Autodesk Fusion 360 part; units mm, degrees
(part 6 of 15)
  spline S62 degree 5 poles (-42.8106, 4.7487) (-42.8188, 4.7555) (-42.8407, 4.7736) (-42.8766, 4.8029) (-42.9264, 4.8435) (-42.9903, 4.8952) (-43.0603, 4.9512) (-43.1305, 5.0069) (-43.2011, 5.0623) (-43.2719, 5.1174) (-43.3431, 5.1723) (-43.4145, 5.2269) (-43.4863, 5.2813) (-43.5583, 5.3354) (-43.6306, 5.3892) (-43.7031, 5.4428) (-43.776, 5.4962) (-43.8491, 5.5492) (-43.9224, 5.6021) (-43.9961, 5.6546) (-44.07, 5.707) (-44.1441, 5.7591) (-44.2185, 5.8109) (-44.2932, 5.8625) (-44.3681, 5.9139) (-44.4432, 5.965) (-44.5186, 6.0159) (-44.5942, 6.0665) (-44.6701, 6.1169) (-44.7462, 6.1671) (-44.8225, 6.2171) (-44.8991, 6.2668) (-44.9758, 6.3163) (-45.0529, 6.3656) (-45.1301, 6.4146) (-45.2075, 6.4634) (-45.2852, 6.512) (-45.3631, 6.5604) (-45.4412, 6.6085) (-45.5196, 6.6564) (-45.5981, 6.7041) (-45.6769, 6.7516) (-45.7558, 6.7988) (-45.8191, 6.8365) (-45.8667, 6.8646) (-45.8985, 6.8833) (-45.9144, 6.8927) knots 0.405839 0.405839 0.405839 0.405839 0.405839 0.405839 0.414286 0.428571 0.442857 0.457143 0.471429 0.485714 0.5 0.514286 0.528571 0.542857 0.557143 0.571429 0.585714 0.6 0.614286 0.628571 0.642857 0.657143 0.671429 0.685714 0.7 0.714286 0.728571 0.742857 0.757143 0.771429 0.785714 0.8 0.814286 0.828571 0.842857 0.857143 0.871429 0.885714 0.9 0.914286 0.928571 0.942857 0.957143 0.971429 0.985714 1 1 1 1 1 1
  arc A63 (-45.9144, 6.8927) -> (-46.9733, 6.0999) centre (-2.0032, -52.8695) ccw
  spline S63 degree 5 poles (-46.9733, 6.0999) (-46.9689, 6.0821) (-46.9599, 6.0463) (-46.9463, 5.9927) (-46.928, 5.9213) (-46.9049, 5.8323) (-46.8816, 5.7433) (-46.8579, 5.6545) (-46.834, 5.5659) (-46.8098, 5.4774) (-46.7854, 5.389) (-46.7606, 5.3008) (-46.7356, 5.2127) (-46.7103, 5.1248) (-46.6848, 5.037) (-46.6589, 4.9494) (-46.6328, 4.8619) (-46.6063, 4.7746) (-46.5796, 4.6875) (-46.5526, 4.6005) (-46.5253, 4.5136) (-46.4977, 4.427) (-46.4699, 4.3405) (-46.4417, 4.2541) (-46.4132, 4.168) (-46.3844, 4.082) (-46.3553, 3.9962) (-46.3259, 3.9105) (-46.2962, 3.8251) (-46.2662, 3.7398) (-46.2359, 3.6547) (-46.2052, 3.5698) (-46.1743, 3.485) (-46.143, 3.4005) (-46.1114, 3.3162) (-46.0794, 3.232) (-46.0471, 3.1481) (-46.0145, 3.0644) (-45.9816, 2.9808) (-45.9483, 2.8975) (-45.9146, 2.8144) (-45.8806, 2.7315) (-45.849, 2.6556) (-45.8241, 2.5964) (-45.806, 2.5537) (-45.7949, 2.5276) (-45.7907, 2.5179) knots -1 -1 -1 -1 -1 -1 -0.985714 -0.971429 -0.957143 -0.942857 -0.928571 -0.914286 -0.9 -0.885714 -0.871429 -0.857143 -0.842857 -0.828571 -0.814286 -0.8 -0.785714 -0.771429 -0.757143 -0.742857 -0.728571 -0.714286 -0.7 -0.685714 -0.671429 -0.657143 -0.642857 -0.628571 -0.614286 -0.6 -0.585714 -0.571429 -0.557143 -0.542857 -0.528571 -0.514286 -0.5 -0.485714 -0.471429 -0.457143 -0.442857 -0.428571 -0.414286 -0.405839 -0.405839 -0.405839 -0.405839 -0.405839 -0.405839
  arc A64 (-45.7907, 2.5179) -> (-46.8171, 1.6908) centre (-2.0032, -52.8695) ccw
  spline S64 degree 5 poles (-46.8171, 1.6908) (-46.8257, 1.6969) (-46.8489, 1.7134) (-46.8867, 1.7401) (-46.9393, 1.7771) (-47.0068, 1.824) (-47.0805, 1.8749) (-47.1546, 1.9254) (-47.2289, 1.9757) (-47.3035, 2.0256) (-47.3784, 2.0753) (-47.4536, 2.1247) (-47.529, 2.1738) (-47.6047, 2.2226) (-47.6806, 2.2711) (-47.7568, 2.3194) (-47.8333, 2.3674) (-47.91, 2.4151) (-47.987, 2.4626) (-48.0641, 2.5098) (-48.1416, 2.5567) (-48.2193, 2.6034) (-48.2972, 2.6498) (-48.3753, 2.6959) (-48.4537, 2.7418) (-48.5323, 2.7874) (-48.6111, 2.8328) (-48.6901, 2.878) (-48.7694, 2.9228) (-48.8489, 2.9675) (-48.9286, 3.0118) (-49.0085, 3.056) (-49.0886, 3.0999) (-49.1689, 3.1435) (-49.2495, 3.1869) (-49.3302, 3.2301) (-49.4112, 3.273) (-49.4923, 3.3157) (-49.5737, 3.3581) (-49.6552, 3.4003) (-49.737, 3.4423) (-49.8189, 3.484) (-49.901, 3.5255) (-49.9669, 3.5586) (-50.0164, 3.5832) (-50.0494, 3.5996) (-50.0659, 3.6078) knots 0.405839 0.405839 0.405839 0.405839 0.405839 0.405839 0.414286 0.428571 0.442857 0.457143 0.471429 0.485714 0.5 0.514286 0.528571 0.542857 0.557143 0.571429 0.585714 0.6 0.614286 0.628571 0.642857 0.657143 0.671429 0.685714 0.7 0.714286 0.728571 0.742857 0.757143 0.771429 0.785714 0.8 0.814286 0.828571 0.842857 0.857143 0.871429 0.885714 0.9 0.914286 0.928571 0.942857 0.957143 0.971429 0.985714 1 1 1 1 1 1
  arc A65 (-50.0659, 3.6078) -> (-51.0656, 2.7416) centre (-2.0032, -52.8695) ccw
  spline S65 degree 5 poles (-51.0656, 2.7416) (-51.0598, 2.724) (-51.0483, 2.689) (-51.031, 2.6365) (-51.0077, 2.5666) (-50.9783, 2.4794) (-50.9486, 2.3924) (-50.9187, 2.3055) (-50.8885, 2.2188) (-50.8581, 2.1322) (-50.8274, 2.0458) (-50.7964, 1.9596) (-50.7652, 1.8735) (-50.7337, 1.7877) (-50.7019, 1.7019) (-50.6699, 1.6164) (-50.6376, 1.531) (-50.605, 1.4458) (-50.5721, 1.3608) (-50.539, 1.2759) (-50.5056, 1.1913) (-50.4719, 1.1068) (-50.4379, 1.0225) (-50.4036, 0.9384) (-50.3691, 0.8545) (-50.3342, 0.7708) (-50.2991, 0.6872) (-50.2636, 0.6039) (-50.2279, 0.5208) (-50.1919, 0.4379) (-50.1556, 0.3551) (-50.1189, 0.2726) (-50.082, 0.1903) (-50.0448, 0.1083) (-50.0072, 0.0264) (-49.9693, -0.0553) (-49.9312, -0.1367) (-49.8927, -0.2179) (-49.8538, -0.2988) (-49.8147, -0.3796) (-49.7752, -0.4601) (-49.7353, -0.5403) (-49.6985, -0.6138) (-49.6694, -0.6711) (-49.6483, -0.7123) (-49.6353, -0.7376) (-49.6305, -0.747) knots -1 -1 -1 -1 -1 -1 -0.985714 -0.971429 -0.957143 -0.942857 -0.928571 -0.914286 -0.9 -0.885714 -0.871429 -0.857143 -0.842857 -0.828571 -0.814286 -0.8 -0.785714 -0.771429 -0.757143 -0.742857 -0.728571 -0.714286 -0.7 -0.685714 -0.671429 -0.657143 -0.642857 -0.628571 -0.614286 -0.6 -0.585714 -0.571429 -0.557143 -0.542857 -0.528571 -0.514286 -0.5 -0.485714 -0.471429 -0.457143 -0.442857 -0.428571 -0.414286 -0.405839 -0.405839 -0.405839 -0.405839 -0.405839 -0.405839
  arc A66 (-49.6305, -0.747) -> (-50.5952, -1.6452) centre (-2.0032, -52.8695) ccw
  spline S66 degree 5 poles (-50.5952, -1.6452) (-50.6042, -1.6397) (-50.6285, -1.625) (-50.6682, -1.601) (-50.7232, -1.5679) (-50.7939, -1.5259) (-50.8711, -1.4804) (-50.9486, -1.4353) (-51.0263, -1.3904) (-51.1043, -1.3459) (-51.1825, -1.3017) (-51.261, -1.2578) (-51.3397, -1.2142) (-51.4187, -1.1709) (-51.4979, -1.1279) (-51.5774, -1.0852) (-51.6571, -1.0428) (-51.737, -1.0007) (-51.8171, -0.9588) (-51.8975, -0.9173) (-51.9781, -0.876) (-52.0589, -0.835) (-52.1399, -0.7942) (-52.2211, -0.7538) (-52.3026, -0.7136) (-52.3842, -0.6737) (-52.4661, -0.6341) (-52.5482, -0.5947) (-52.6304, -0.5556) (-52.7129, -0.5167) (-52.7955, -0.4782) (-52.8784, -0.4398) (-52.9615, -0.4018) (-53.0447, -0.364) (-53.1281, -0.3264) (-53.2117, -0.2891) (-53.2955, -0.2521) (-53.3795, -0.2153) (-53.4637, -0.1788) (-53.548, -0.1425) (-53.6326, -0.1065) (-53.7173, -0.0707) (-53.8022, -0.0351) (-53.8702, -0.0069) (-53.9213, 0.0142) (-53.9554, 0.0282) (-53.9725, 0.0351) knots 0.405839 0.405839 0.405839 0.405839 0.405839 0.405839 0.414286 0.428571 0.442857 0.457143 0.471429 0.485714 0.5 0.514286 0.528571 0.542857 0.557143 0.571429 0.585714 0.6 0.614286 0.628571 0.642857 0.657143 0.671429 0.685714 0.7 0.714286 0.728571 0.742857 0.757143 0.771429 0.785714 0.8 0.814286 0.828571 0.842857 0.857143 0.871429 0.885714 0.9 0.914286 0.928571 0.942857 0.957143 0.971429 0.985714 1 1 1 1 1 1
  arc A67 (-53.9725, 0.0351) -> (-54.9078, -0.9002) centre (-2.0032, -52.8695) ccw
  spline S67 degree 5 poles (-54.9078, -0.9002) (-54.9009, -0.9173) (-54.8869, -0.9514) (-54.8658, -1.0025) (-54.8376, -1.0705) (-54.802, -1.1554) (-54.7662, -1.2401) (-54.7302, -1.3246) (-54.6939, -1.409) (-54.6574, -1.4932) (-54.6206, -1.5772) (-54.5836, -1.661) (-54.5463, -1.7446) (-54.5087, -1.828) (-54.4709, -1.9112) (-54.4329, -1.9943) (-54.3945, -2.0771) (-54.356, -2.1598) (-54.3171, -2.2423) (-54.278, -2.3245) (-54.2386, -2.4066) (-54.199, -2.4885) (-54.1591, -2.5701) (-54.1189, -2.6515) (-54.0784, -2.7328) (-54.0377, -2.8138) (-53.9967, -2.8946) (-53.9554, -2.9752) (-53.9139, -3.0556) (-53.872, -3.1357) (-53.8299, -3.2156) (-53.7875, -3.2953) (-53.7448, -3.3748) (-53.7018, -3.454) (-53.6585, -3.533) (-53.6149, -3.6117) (-53.571, -3.6902) (-53.5268, -3.7684) (-53.4822, -3.8464) (-53.4374, -3.9241) (-53.3923, -4.0016) (-53.3468, -4.0788) (-53.3048, -4.1495) (-53.2717, -4.2045) (-53.2477, -4.2442) (-53.233, -4.2685) (-53.2275, -4.2775) knots -1 -1 -1 -1 -1 -1 -0.985714 -0.971429 -0.957143 -0.942857 -0.928571 -0.914286 -0.9 -0.885714 -0.871429 -0.857143 -0.842857 -0.828571 -0.814286 -0.8 -0.785714 -0.771429 -0.757143 -0.742857 -0.728571 -0.714286 -0.7 -0.685714 -0.671429 -0.657143 -0.642857 -0.628571 -0.614286 -0.6 -0.585714 -0.571429 -0.557143 -0.542857 -0.528571 -0.514286 -0.5 -0.485714 -0.471429 -0.457143 -0.442857 -0.428571 -0.414286 -0.405839 -0.405839 -0.405839 -0.405839 -0.405839 -0.405839
  arc A68 (-53.2275, -4.2775) -> (-54.1257, -5.2422) centre (-2.0032, -52.8695) ccw
  spline S68 degree 5 poles (-54.1257, -5.2422) (-54.1351, -5.2374) (-54.1604, -5.2244) (-54.2016, -5.2033) (-54.2589, -5.1742) (-54.3324, -5.1374) (-54.4126, -5.0975) (-54.4931, -5.058) (-54.5739, -5.0189) (-54.6548, -4.98) (-54.736, -4.9415) (-54.8174, -4.9033) (-54.8991, -4.8655) (-54.9809, -4.8279) (-55.063, -4.7907) (-55.1453, -4.7538) (-55.2278, -4.7171) (-55.3106, -4.6808) (-55.3935, -4.6448) (-55.4766, -4.6091) (-55.5599, -4.5736) (-55.6435, -4.5385) (-55.7272, -4.5036) (-55.8111, -4.4691) (-55.8952, -4.4348) (-55.9795, -4.4008) (-56.064, -4.3671) (-56.1486, -4.3337) (-56.2335, -4.3006) (-56.3185, -4.2677) (-56.4037, -4.2351) (-56.4891, -4.2028) (-56.5746, -4.1708) (-56.6603, -4.139) (-56.7462, -4.1075) (-56.8323, -4.0763) (-56.9185, -4.0453) (-57.0049, -4.0146) (-57.0915, -3.9842) (-57.1782, -3.954) (-57.2651, -3.9241) (-57.3521, -3.8944) (-57.4393, -3.865) (-57.5092, -3.8417) (-57.5617, -3.8244) (-57.5967, -3.8128) (-57.6143, -3.8071) knots 0.405839 0.405839 0.405839 0.405839 0.405839 0.405839 0.414286 0.428571 0.442857 0.457143 0.471429 0.485714 0.5 0.514286 0.528571 0.542857 0.557143 0.571429 0.585714 0.6 0.614286 0.628571 0.642857 0.657143 0.671429 0.685714 0.7 0.714286 0.728571 0.742857 0.757143 0.771429 0.785714 0.8 0.814286 0.828571 0.842857 0.857143 0.871429 0.885714 0.9 0.914286 0.928571 0.942857 0.957143 0.971429 0.985714 1 1 1 1 1 1
  arc A69 (-57.6143, -3.8071) -> (-58.4805, -4.8068) centre (-2.0032, -52.8695) ccw
  spline S69 degree 5 poles (-58.4805, -4.8068) (-58.4723, -4.8233) (-58.4559, -4.8563) (-58.4313, -4.9058) (-58.3982, -4.9717) (-58.3567, -5.0538) (-58.315, -5.1357) (-58.273, -5.2175) (-58.2308, -5.299) (-58.1884, -5.3804) (-58.1457, -5.4615) (-58.1028, -5.5425) (-58.0596, -5.6232) (-58.0162, -5.7037) (-57.9726, -5.7841) (-57.9287, -5.8642) (-57.8845, -5.9441) (-57.8402, -6.0238) (-57.7955, -6.1033) (-57.7507, -6.1826) (-57.7055, -6.2616) (-57.6601, -6.3404) (-57.6145, -6.419) (-57.5686, -6.4974) (-57.5225, -6.5755) (-57.4761, -6.6534) (-57.4294, -6.7311) (-57.3825, -6.8085) (-57.3353, -6.8857) (-57.2878, -6.9627) (-57.2401, -7.0394) (-57.1921, -7.1159) (-57.1438, -7.1921) (-57.0953, -7.268) (-57.0465, -7.3437) (-56.9974, -7.4191) (-56.948, -7.4943) (-56.8983, -7.5692) (-56.8484, -7.6438) (-56.7981, -7.7181) (-56.7476, -7.7922) (-56.6967, -7.8659) (-56.6497, -7.9334) (-56.6128, -7.986) (-56.5861, -8.0238) (-56.5696, -8.047) (-56.5635, -8.0556) knots -1 -1 -1 -1 -1 -1 -0.985714 -0.971429 -0.957143 -0.942857 -0.928571 -0.914286 -0.9 -0.885714 -0.871429 -0.857143 -0.842857 -0.828571 -0.814286 -0.8 -0.785714 -0.771429 -0.757143 -0.742857 -0.728571 -0.714286 -0.7 -0.685714 -0.671429 -0.657143 -0.642857 -0.628571 -0.614286 -0.6 -0.585714 -0.571429 -0.557143 -0.542857 -0.528571 -0.514286 -0.5 -0.485714 -0.471429 -0.457143 -0.442857 -0.428571 -0.414286 -0.405839 -0.405839 -0.405839 -0.405839 -0.405839 -0.405839
  arc A70 (-56.5635, -8.0556) -> (-57.3905, -9.082) centre (-2.0032, -52.8695) ccw
  spline S70 degree 5 poles (-57.3905, -9.082) (-57.4003, -9.0778) (-57.4264, -9.0667) (-57.4691, -9.0486) (-57.5283, -9.0236) (-57.6042, -8.9921) (-57.6871, -8.9581) (-57.7702, -8.9244) (-57.8535, -8.8911) (-57.9371, -8.8582) (-58.0208, -8.8256) (-58.1047, -8.7933) (-58.1889, -8.7613) (-58.2732, -8.7297) (-58.3577, -8.6984) (-58.4425, -8.6675) (-58.5274, -8.6368) (-58.6125, -8.6065) (-58.6978, -8.5765) (-58.7832, -8.5468) (-58.8689, -8.5174) (-58.9547, -8.4883) (-59.0407, -8.4595) (-59.1268, -8.431) (-59.2132, -8.4028) (-59.2997, -8.3749) (-59.3863, -8.3474) (-59.4732, -8.3201) (-59.5602, -8.2931) (-59.6473, -8.2664) (-59.7346, -8.2399) (-59.8221, -8.2138) (-59.9097, -8.1879) (-59.9975, -8.1624) (-60.0854, -8.1371) (-60.1735, -8.1121) (-60.2617, -8.0873) (-60.3501, -8.0629) (-60.4386, -8.0387) (-60.5272, -8.0148) (-60.616, -7.9911) (-60.705, -7.9678) (-60.794, -7.9447) (-60.8654, -7.9264) (-60.919, -7.9128) (-60.9548, -7.9038) (-60.9726, -7.8993) knots 0.405839 0.405839 0.405839 0.405839 0.405839 0.405839 0.414286 0.428571 0.442857 0.457143 0.471429 0.485714 0.5 0.514286 0.528571 0.542857 0.557143 0.571429 0.585714 0.6 0.614286 0.628571 0.642857 0.657143 0.671429 0.685714 0.7 0.714286 0.728571 0.742857 0.757143 0.771429 0.785714 0.8 0.814286 0.828571 0.842857 0.857143 0.871429 0.885714 0.9 0.914286 0.928571 0.942857 0.957143 0.971429 0.985714 1 1 1 1 1 1
  arc A71 (-60.9726, -7.8993) -> (-61.7653, -8.9583) centre (-2.0032, -52.8695) ccw
  spline S71 degree 5 poles (-61.7653, -8.9583) (-61.756, -8.9742) (-61.7373, -9.006) (-61.7092, -9.0535) (-61.6715, -9.1169) (-61.6243, -9.1958) (-61.5768, -9.2746) (-61.5291, -9.3531) (-61.4812, -9.4315) (-61.4331, -9.5096) (-61.3847, -9.5875) (-61.3361, -9.6651) (-61.2873, -9.7426) (-61.2383, -9.8198) (-61.189, -9.8969) (-61.1395, -9.9736) (-61.0898, -10.0502) (-61.0398, -10.1265) (-60.9896, -10.2026) (-60.9392, -10.2785) (-60.8886, -10.3541) (-60.8377, -10.4295) (-60.7866, -10.5046) (-60.7352, -10.5795) (-60.6836, -10.6542) (-60.6317, -10.7286) (-60.5797, -10.8027) (-60.5273, -10.8766) (-60.4747, -10.9502) (-60.4219, -11.0236) (-60.3688, -11.0967) (-60.3155, -11.1696) (-60.2619, -11.2421) (-60.2081, -11.3144) (-60.154, -11.3864) (-60.0996, -11.4582) (-60.045, -11.5296) (-59.9901, -11.6008) (-59.935, -11.6716) (-59.8795, -11.7422) (-59.8238, -11.8124) (-59.7679, -11.8824) (-59.7162, -11.9463) (-59.6756, -11.9961) (-59.6462, -12.032) (-59.6282, -12.0539) (-59.6214, -12.0621) knots -1 -1 -1 -1 -1 -1 -0.985714 -0.971429 -0.957143 -0.942857 -0.928571 -0.914286 -0.9 -0.885714 -0.871429 -0.857143 -0.842857 -0.828571 -0.814286 -0.8 -0.785714 -0.771429 -0.757143 -0.742857 -0.728571 -0.714286 -0.7 -0.685714 -0.671429 -0.657143 -0.642857 -0.628571 -0.614286 -0.6 -0.585714 -0.571429 -0.557143 -0.542857 -0.528571 -0.514286 -0.5 -0.485714 -0.471429 -0.457143 -0.442857 -0.428571 -0.414286 -0.405839 -0.405839 -0.405839 -0.405839 -0.405839 -0.405839
  arc A72 (-59.6214, -12.0621) -> (-60.3732, -13.1448) centre (-2.0032, -52.8695) ccw
  spline S72 degree 5 poles (-60.3732, -13.1448) (-60.3832, -13.1414) (-60.4101, -13.1321) (-60.4539, -13.1171) (-60.5148, -13.0965) (-60.5927, -13.0704) (-60.6778, -13.0424) (-60.7631, -13.0148) (-60.8486, -12.9875) (-60.9343, -12.9606) (-61.0201, -12.934) (-61.1062, -12.9078) (-61.1924, -12.882) (-61.2787, -12.8564) (-61.3653, -12.8313) (-61.452, -12.8064) (-61.5389, -12.7819) (-61.6259, -12.7577) (-61.7131, -12.7339) (-61.8005, -12.7103) (-61.888, -12.6871) (-61.9757, -12.6642) (-62.0635, -12.6417) (-62.1515, -12.6194) (-62.2396, -12.5974) (-62.3279, -12.5758) (-62.4163, -12.5545) (-62.5049, -12.5334) (-62.5936, -12.5127) (-62.6824, -12.4923) (-62.7714, -12.4721) (-62.8605, -12.4523) (-62.9497, -12.4328) (-63.0391, -12.4135) (-63.1286, -12.3946) (-63.2182, -12.3759) (-63.308, -12.3575) (-63.3979, -12.3394) (-63.4879, -12.3216) (-63.578, -12.3041) (-63.6683, -12.2869) (-63.7586, -12.2699) (-63.8491, -12.2532) (-63.9216, -12.2401) (-63.9761, -12.2304) (-64.0124, -12.224) (-64.0305, -12.2208) knots 0.405839 0.405839 0.405839 0.405839 0.405839 0.405839 0.414286 0.428571 0.442857 0.457143 0.471429 0.485714 0.5 0.514286 0.528571 0.542857 0.557143 0.571429 0.585714 0.6 0.614286 0.628571 0.642857 0.657143 0.671429 0.685714 0.7 0.714286 0.728571 0.742857 0.757143 0.771429 0.785714 0.8 0.814286 0.828571 0.842857 0.857143 0.871429 0.885714 0.9 0.914286 0.928571 0.942857 0.957143 0.971429 0.985714 1 1 1 1 1 1
  arc A73 (-64.0305, -12.2208) -> (-64.7457, -13.3335) centre (-2.0032, -52.8695) ccw
  spline S73 degree 5 poles (-64.7457, -13.3335) (-64.7352, -13.3487) (-64.7143, -13.3791) (-64.6828, -13.4246) (-64.6408, -13.485) (-64.588, -13.5604) (-64.535, -13.6356) (-64.4819, -13.7105) (-64.4285, -13.7852) (-64.3749, -13.8597) (-64.3211, -13.934) (-64.2671, -14.008) (-64.2129, -14.0818) (-64.1585, -14.1553) (-64.1038, -14.2286) (-64.049, -14.3017) (-63.9939, -14.3745) (-63.9386, -14.4471) (-63.8832, -14.5194) (-63.8275, -14.5914) (-63.7715, -14.6633) (-63.7154, -14.7348) (-63.6591, -14.8061) (-63.6025, -14.8772) (-63.5457, -14.9479) (-63.4887, -15.0185) (-63.4314, -15.0887) (-63.374, -15.1587) (-63.3163, -15.2284) (-63.2583, -15.2978) (-63.2002, -15.3669) (-63.1418, -15.4358) (-63.0832, -15.5043) (-63.0243, -15.5726) (-62.9652, -15.6406) (-62.9059, -15.7082) (-62.8463, -15.7756) (-62.7865, -15.8427) (-62.7264, -15.9094) (-62.6661, -15.9758) (-62.6055, -16.0419) (-62.5447, -16.1077) (-62.4886, -16.1678) (-62.4446, -16.2146) (-62.4127, -16.2482) (-62.3931, -16.2688) (-62.3858, -16.2765) knots -1 -1 -1 -1 -1 -1 -0.985714 -0.971429 -0.957143 -0.942857 -0.928571 -0.914286 -0.9 -0.885714 -0.871429 -0.857143 -0.842857 -0.828571 -0.814286 -0.8 -0.785714 -0.771429 -0.757143 -0.742857 -0.728571 -0.714286 -0.7 -0.685714 -0.671429 -0.657143 -0.642857 -0.628571 -0.614286 -0.6 -0.585714 -0.571429 -0.557143 -0.542857 -0.528571 -0.514286 -0.5 -0.485714 -0.471429 -0.457143 -0.442857 -0.428571 -0.414286 -0.405839 -0.405839 -0.405839 -0.405839 -0.405839 -0.405839
  arc A74 (-62.3858, -16.2765) -> (-63.0584, -17.4101) centre (-2.0032, -52.8695) ccw
  spline S74 degree 5 poles (-63.0584, -17.4101) (-63.0686, -17.4074) (-63.0961, -17.4) (-63.1409, -17.3882) (-63.2031, -17.372) (-63.2827, -17.3516) (-63.3696, -17.3297) (-63.4566, -17.3082) (-63.5438, -17.2871) (-63.6312, -17.2664) (-63.7187, -17.246) (-63.8064, -17.226) (-63.8942, -17.2063) (-63.9822, -17.1871) (-64.0703, -17.1681) (-64.1586, -17.1495) (-64.247, -17.1313) (-64.3356, -17.1134) (-64.4242, -17.0958) (-64.5131, -17.0785) (-64.602, -17.0616) (-64.6911, -17.0451) (-64.7803, -17.0288) (-64.8697, -17.0129) (-64.9591, -16.9973) (-65.0487, -16.982) (-65.1384, -16.967) (-65.2282, -16.9523) (-65.3182, -16.938) (-65.4083, -16.924) (-65.4984, -16.9102) (-65.5887, -16.8968) (-65.6791, -16.8837) (-65.7697, -16.8709) (-65.8603, -16.8583) (-65.951, -16.8461) (-66.0419, -16.8342) (-66.1328, -16.8226) (-66.2239, -16.8112) (-66.315, -16.8002) (-66.4063, -16.7894) (-66.4976, -16.7789) (-66.5891, -16.7687) (-66.6623, -16.7608) (-66.7173, -16.755) (-66.754, -16.7512) (-66.7723, -16.7493) knots 0.405839 0.405839 0.405839 0.405839 0.405839 0.405839 0.414286 0.428571 0.442857 0.457143 0.471429 0.485714 0.5 0.514286 0.528571 0.542857 0.557143 0.571429 0.585714 0.6 0.614286 0.628571 0.642857 0.657143 0.671429 0.685714 0.7 0.714286 0.728571 0.742857 0.757143 0.771429 0.785714 0.8 0.814286 0.828571 0.842857 0.857143 0.871429 0.885714 0.9 0.914286 0.928571 0.942857 0.957143 0.971429 0.985714 1 1 1 1 1 1
  arc A75 (-66.7723, -16.7493) -> (-67.4063, -17.9103) centre (-2.0032, -52.8695) ccw
  spline S75 degree 5 poles (-67.4063, -17.9103) (-67.3948, -17.9247) (-67.3717, -17.9535) (-67.3371, -17.9966) (-67.2908, -18.0539) (-67.2328, -18.1253) (-67.1746, -18.1965) (-67.1162, -18.2675) (-67.0577, -18.3382) (-66.9989, -18.4087) (-66.9399, -18.4789) (-66.8808, -18.5489) (-66.8215, -18.6186) (-66.7619, -18.6881) (-66.7022, -18.7573) (-66.6423, -18.8262) (-66.5822, -18.8949) (-66.5219, -18.9634) (-66.4614, -19.0316) (-66.4007, -19.0995) (-66.3398, -19.1671) (-66.2787, -19.2345) (-66.2174, -19.3016) (-66.1559, -19.3684) (-66.0942, -19.435) (-66.0323, -19.5012) (-65.9702, -19.5672) (-65.9078, -19.6329) (-65.8453, -19.6983) (-65.7826, -19.7634) (-65.7197, -19.8282) (-65.6565, -19.8927) (-65.5931, -19.9569) (-65.5296, -20.0208) (-65.4658, -20.0844) (-65.4017, -20.1477) (-65.3375, -20.2106) (-65.2731, -20.2732) (-65.2084, -20.3355) (-65.1435, -20.3975) (-65.0783, -20.4591) (-65.013, -20.5203) (-64.9528, -20.5763) (-64.9055, -20.6198) (-64.8713, -20.6511) (-64.8503, -20.6703) (-64.8425, -20.6774) knots -1 -1 -1 -1 -1 -1 -0.985714 -0.971429 -0.957143 -0.942857 -0.928571 -0.914286 -0.9 -0.885714 -0.871429 -0.857143 -0.842857 -0.828571 -0.814286 -0.8 -0.785714 -0.771429 -0.757143 -0.742857 -0.728571 -0.714286 -0.7 -0.685714 -0.671429 -0.657143 -0.642857 -0.628571 -0.614286 -0.6 -0.585714 -0.571429 -0.557143 -0.542857 -0.528571 -0.514286 -0.5 -0.485714 -0.471429 -0.457143 -0.442857 -0.428571 -0.414286 -0.405839 -0.405839 -0.405839 -0.405839 -0.405839 -0.405839
  arc A76 (-64.8425, -20.6774) -> (-65.4325, -21.8561) centre (-2.0032, -52.8695) ccw
  spline S76 degree 5 poles (-65.4325, -21.8561) (-65.4429, -21.8541) (-65.4708, -21.8487) (-65.5163, -21.8401) (-65.5795, -21.8284) (-65.6604, -21.8137) (-65.7486, -21.7981) (-65.837, -21.7829) (-65.9254, -21.768) (-66.0141, -21.7536) (-66.1028, -21.7395) (-66.1917, -21.7258) (-66.2807, -21.7125) (-66.3698, -21.6995) (-66.4591, -21.6869) (-66.5485, -21.6746) (-66.638, -21.6627) (-66.7276, -21.6512) (-66.8173, -21.64) (-66.9071, -21.6291) (-66.997, -21.6186) (-67.0871, -21.6084) (-67.1772, -21.5986) (-67.2675, -21.5891) (-67.3578, -21.5799) (-67.4483, -21.571) (-67.5388, -21.5625) (-67.6295, -21.5543) (-67.7202, -21.5464) (-67.811, -21.5388) (-67.902, -21.5315) (-67.993, -21.5246) (-68.0841, -21.518) (-68.1753, -21.5116) (-68.2666, -21.5056) (-68.358, -21.4999) (-68.4494, -21.4945) (-68.541, -21.4894) (-68.6326, -21.4845) (-68.7243, -21.48) (-68.8161, -21.4758) (-68.908, -21.4719) (-68.9999, -21.4682) (-69.0736, -21.4656) (-69.1288, -21.4637) (-69.1657, -21.4625) (-69.1841, -21.4619) knots 0.405839 0.405839 0.405839 0.405839 0.405839 0.405839 0.414286 0.428571 0.442857 0.457143 0.471429 0.485714 0.5 0.514286 0.528571 0.542857 0.557143 0.571429 0.585714 0.6 0.614286 0.628571 0.642857 0.657143 0.671429 0.685714 0.7 0.714286 0.728571 0.742857 0.757143 0.771429 0.785714 0.8 0.814286 0.828571 0.842857 0.857143 0.871429 0.885714 0.9 0.914286 0.928571 0.942857 0.957143 0.971429 0.985714 1 1 1 1 1 1
  arc A77 (-69.1841, -21.4619) -> (-69.7336, -22.6651) centre (-2.0032, -52.8695) ccw
  spline S77 degree 5 poles (-69.7336, -22.6651) (-69.7211, -22.6787) (-69.6961, -22.7058) (-69.6585, -22.7463) (-69.6082, -22.8002) (-69.5453, -22.8673) (-69.4821, -22.9341) (-69.4188, -23.0008) (-69.3553, -23.0671) (-69.2917, -23.1332) (-69.2279, -23.199) (-69.1639, -23.2646) (-69.0997, -23.3299) (-69.0354, -23.395) (-68.9709, -23.4598) (-68.9062, -23.5243) (-68.8414, -23.5885) (-68.7763, -23.6525) (-68.7111, -23.7162) (-68.6457, -23.7796) (-68.5801, -23.8427) (-68.5144, -23.9055) (-68.4485, -23.9681) (-68.3824, -24.0304) (-68.3161, -24.0923) (-68.2496, -24.154) (-68.1829, -24.2154) (-68.1161, -24.2765) (-68.0491, -24.3373) (-67.9818, -24.3977) (-67.9144, -24.4579) (-67.8469, -24.5177) (-67.7791, -24.5772) (-67.7111, -24.6364) (-67.6429, -24.6953) (-67.5746, -24.7538) (-67.506, -24.812) (-67.4372, -24.8699) (-67.3683, -24.9274) (-67.2991, -24.9846) (-67.2298, -25.0414) (-67.1602, -25.0978) (-67.0961, -25.1493) (-67.0459, -25.1894) (-67.0096, -25.2181) (-66.9872, -25.2358) (-66.9789, -25.2423) knots -1 -1 -1 -1 -1 -1 -0.985714 -0.971429 -0.957143 -0.942857 -0.928571 -0.914286 -0.9 -0.885714 -0.871429 -0.857143 -0.842857 -0.828571 -0.814286 -0.8 -0.785714 -0.771429 -0.757143 -0.742857 -0.728571 -0.714286 -0.7 -0.685714 -0.671429 -0.657143 -0.642857 -0.628571 -0.614286 -0.6 -0.585714 -0.571429 -0.557143 -0.542857 -0.528571 -0.514286 -0.5 -0.485714 -0.471429 -0.457143 -0.442857 -0.428571 -0.414286 -0.405839 -0.405839 -0.405839 -0.405839 -0.405839 -0.405839
  arc A78 (-66.9789, -25.2423) -> (-67.4833, -26.4601) centre (-2.0032, -52.8695) ccw
  spline S78 degree 5 poles (-67.4833, -26.4601) (-67.4938, -26.4588) (-67.5221, -26.4555) (-67.5681, -26.4502) (-67.632, -26.4429) (-67.7137, -26.4341) (-67.8028, -26.4248) (-67.892, -26.4159) (-67.9813, -26.4074) (-68.0708, -26.3993) (-68.1603, -26.3916) (-68.2499, -26.3843) (-68.3397, -26.3774) (-68.4295, -26.3708) (-68.5194, -26.3646) (-68.6094, -26.3587) (-68.6995, -26.3532) (-68.7897, -26.3481) (-68.88, -26.3433) (-68.9704, -26.3389) (-69.0608, -26.3348) (-69.1514, -26.3311) (-69.242, -26.3277) (-69.3327, -26.3247) (-69.4235, -26.322) (-69.5143, -26.3196) (-69.6052, -26.3175) (-69.6962, -26.3158) (-69.7873, -26.3144) (-69.8785, -26.3133) (-69.9697, -26.3126) (-70.061, -26.3121) (-70.1523, -26.312) (-70.2438, -26.3122) (-70.3352, -26.3127) (-70.4268, -26.3135) (-70.5184, -26.3146) (-70.6101, -26.3161) (-70.7018, -26.3178) (-70.7936, -26.3198) (-70.8855, -26.3222) (-70.9774, -26.3248) (-71.0694, -26.3277) (-71.143, -26.3303) (-71.1982, -26.3324) (-71.2351, -26.3338) (-71.2535, -26.3346) knots 0.405839 0.405839 0.405839 0.405839 0.405839 0.405839 0.414286 0.428571 0.442857 0.457143 0.471429 0.485714 0.5 0.514286 0.528571 0.542857 0.557143 0.571429 0.585714 0.6 0.614286 0.628571 0.642857 0.657143 0.671429 0.685714 0.7 0.714286 0.728571 0.742857 0.757143 0.771429 0.785714 0.8 0.814286 0.828571 0.842857 0.857143 0.871429 0.885714 0.9 0.914286 0.928571 0.942857 0.957143 0.971429 0.985714 1 1 1 1 1 1
  arc A79 (-71.2535, -26.3346) -> (-71.7158, -27.5739) centre (-2.0032, -52.8695) ccw
  spline S79 degree 5 poles (-71.7158, -27.5739) (-71.7023, -27.5866) (-71.6754, -27.6118) (-71.635, -27.6495) (-71.5811, -27.6997) (-71.5135, -27.7621) (-71.4458, -27.8243) (-71.3779, -27.8862) (-71.3098, -27.9479) (-71.2416, -28.0093) (-71.1733, -28.0704) (-71.1048, -28.1312) (-71.0361, -28.1918) (-70.9673, -28.2521) (-70.8983, -28.3121) (-70.8292, -28.3718) (-70.7599, -28.4313) (-70.6905, -28.4905) (-70.6209, -28.5493) (-70.5512, -28.6079) (-70.4813, -28.6662) (-70.4112, -28.7242) (-70.341, -28.7819) (-70.2706, -28.8393) (-70.2, -28.8964) (-70.1293, -28.9531) (-70.0585, -29.0096) (-69.9874, -29.0658) (-69.9163, -29.1216) (-69.8449, -29.1771) (-69.7734, -29.2323) (-69.7017, -29.2872) (-69.6298, -29.3417) (-69.5578, -29.3959) (-69.4856, -29.4498) (-69.4132, -29.5033) (-69.3407, -29.5564) (-69.268, -29.6092) (-69.1951, -29.6617) (-69.1221, -29.7138) (-69.0488, -29.7655) (-68.9754, -29.8168) (-68.9078, -29.8636) (-68.8548, -29.9) (-68.8166, -29.9261) (-68.793, -29.9421) (-68.7843, -29.948) knots -1 -1 -1 -1 -1 -1 -0.985714 -0.971429 -0.957143 -0.942857 -0.928571 -0.914286 -0.9 -0.885714 -0.871429 -0.857143 -0.842857 -0.828571 -0.814286 -0.8 -0.785714 -0.771429 -0.757143 -0.742857 -0.728571 -0.714286 -0.7 -0.685714 -0.671429 -0.657143 -0.642857 -0.628571 -0.614286 -0.6 -0.585714 -0.571429 -0.557143 -0.542857 -0.528571 -0.514286 -0.5 -0.485714 -0.471429 -0.457143 -0.442857 -0.428571 -0.414286 -0.405839 -0.405839 -0.405839 -0.405839 -0.405839 -0.405839
  arc A80 (-68.7843, -29.948) -> (-69.2005, -31.1987) centre (-2.0032, -52.8695) ccw
  spline S80 degree 5 poles (-69.2005, -31.1987) (-69.2111, -31.1982) (-69.2395, -31.1969) (-69.2858, -31.1948) (-69.35, -31.1922) (-69.4321, -31.1891) (-69.5217, -31.1862) (-69.6113, -31.1838) (-69.701, -31.1817) (-69.7908, -31.18) (-69.8806, -31.1787) (-69.9706, -31.1778) (-70.0606, -31.1772) (-70.1506, -31.1771) (-70.2408, -31.1773) (-70.331, -31.1779) (-70.4212, -31.1789) (-70.5116, -31.1802) (-70.602, -31.1819) (-70.6924, -31.1839) (-70.7829, -31.1863) (-70.8735, -31.189) (-70.9641, -31.1921) (-71.0548, -31.1955) (-71.1456, -31.1993) (-71.2364, -31.2034) (-71.3272, -31.2078) (-71.4181, -31.2126) (-71.509, -31.2177) (-71.6, -31.2231) (-71.6911, -31.2289) (-71.7822, -31.235) (-71.8733, -31.2414) (-71.9645, -31.2481) (-72.0557, -31.2551) (-72.1469, -31.2624) (-72.2382, -31.2701) (-72.3296, -31.2781) (-72.421, -31.2863) (-72.5124, -31.2949) (-72.6038, -31.3038) (-72.6953, -31.313) (-72.7869, -31.3225) (-72.8601, -31.3303) (-72.9151, -31.3363) (-72.9517, -31.3404) (-72.97, -31.3424) knots 0.405839 0.405839 0.405839 0.405839 0.405839 0.405839 0.414286 0.428571 0.442857 0.457143 0.471429 0.485714 0.5 0.514286 0.528571 0.542857 0.557143 0.571429 0.585714 0.6 0.614286 0.628571 0.642857 0.657143 0.671429 0.685714 0.7 0.714286 0.728571 0.742857 0.757143 0.771429 0.785714 0.8 0.814286 0.828571 0.842857 0.857143 0.871429 0.885714 0.9 0.914286 0.928571 0.942857 0.957143 0.971429 0.985714 1 1 1 1 1 1
  arc A81 (-72.97, -31.3424) -> (-73.3427, -32.6116) centre (-2.0032, -52.8695) ccw
  spline S81 degree 5 poles (-73.3427, -32.6116) (-73.3284, -32.6233) (-73.2998, -32.6465) (-73.2568, -32.6812) (-73.1994, -32.7274) (-73.1275, -32.7849) (-73.0555, -32.8421) (-72.9834, -32.899) (-72.9111, -32.9557) (-72.8387, -33.012) (-72.7662, -33.0681) (-72.6935, -33.1239) (-72.6207, -33.1794) (-72.5478, -33.2347) (-72.4747, -33.2896) (-72.4015, -33.3442) (-72.3282, -33.3986) (-72.2547, -33.4527) (-72.1811, -33.5064) (-72.1073, -33.5599) (-72.0334, -33.613) (-71.9594, -33.6659) (-71.8852, -33.7184) (-71.8109, -33.7706) (-71.7365, -33.8226) (-71.6619, -33.8741) (-71.5872, -33.9254) (-71.5124, -33.9764) (-71.4374, -34.027) (-71.3622, -34.0773) (-71.287, -34.1272) (-71.2115, -34.1768) (-71.136, -34.2261) (-71.0603, -34.275) (-70.9844, -34.3236) (-70.9084, -34.3718) (-70.8323, -34.4196) (-70.756, -34.4671) (-70.6795, -34.5142) (-70.6029, -34.561) (-70.5262, -34.6073) (-70.4493, -34.6533) (-70.3786, -34.6952) (-70.3231, -34.7277) (-70.2831, -34.751) (-70.2585, -34.7652) (-70.2493, -34.7705) knots -1 -1 -1 -1 -1 -1 -0.985714 -0.971429 -0.957143 -0.942857 -0.928571 -0.914286 -0.9 -0.885714 -0.871429 -0.857143 -0.842857 -0.828571 -0.814286 -0.8 -0.785714 -0.771429 -0.757143 -0.742857 -0.728571 -0.714286 -0.7 -0.685714 -0.671429 -0.657143 -0.642857 -0.628571 -0.614286 -0.6 -0.585714 -0.571429 -0.557143 -0.542857 -0.528571 -0.514286 -0.5 -0.485714 -0.471429 -0.457143 -0.442857 -0.428571 -0.414286 -0.405839 -0.405839 -0.405839 -0.405839 -0.405839 -0.405839
  arc A82 (-70.2493, -34.7705) -> (-70.5753, -36.0477) centre (-2.0032, -52.8695) ccw
  spline S82 degree 5 poles (-70.5753, -36.0477) (-70.5859, -36.0479) (-70.6143, -36.0487) (-70.6606, -36.0499) (-70.7248, -36.0519) (-70.807, -36.0547) (-70.8965, -36.0582) (-70.9861, -36.0621) (-71.0757, -36.0664) (-71.1654, -36.0712) (-71.2551, -36.0763) (-71.3449, -36.0818) (-71.4347, -36.0877) (-71.5245, -36.0939) (-71.6144, -36.1006) (-71.7043, -36.1076) (-71.7943, -36.115) (-71.8843, -36.1228) (-71.9744, -36.1309) (-72.0644, -36.1394) (-72.1546, -36.1482) (-72.2447, -36.1574) (-72.3349, -36.167) (-72.4251, -36.1768) (-72.5153, -36.1871) (-72.6056, -36.1976) (-72.6959, -36.2085) (-72.7862, -36.2198) (-72.8766, -36.2314) (-72.9669, -36.2433) (-73.0573, -36.2555) (-73.1478, -36.2681) (-73.2382, -36.2809) (-73.3287, -36.2941) (-73.4191, -36.3077) (-73.5096, -36.3215) (-73.6002, -36.3356) (-73.6907, -36.3501) (-73.7813, -36.3649) (-73.8718, -36.38) (-73.9624, -36.3953) (-74.053, -36.411) (-74.1437, -36.427) (-74.2162, -36.4401) (-74.2706, -36.45) (-74.3068, -36.4566) (-74.325, -36.46) knots 0.405839 0.405839 0.405839 0.405839 0.405839 0.405839 0.414286 0.428571 0.442857 0.457143 0.471429 0.485714 0.5 0.514286 0.528571 0.542857 0.557143 0.571429 0.585714 0.6 0.614286 0.628571 0.642857 0.657143 0.671429 0.685714 0.7 0.714286 0.728571 0.742857 0.757143 0.771429 0.785714 0.8 0.814286 0.828571 0.842857 0.857143 0.871429 0.885714 0.9 0.914286 0.928571 0.942857 0.957143 0.971429 0.985714 1 1 1 1 1 1
  arc A83 (-74.325, -36.46) -> (-74.6061, -37.7525) centre (-2.0032, -52.8695) ccw
  spline S83 degree 5 poles (-74.6061, -37.7525) (-74.591, -37.7631) (-74.5608, -37.7842) (-74.5155, -37.8159) (-74.4549, -37.8578) (-74.3791, -37.91) (-74.3032, -37.9619) (-74.2272, -38.0136) (-74.1511, -38.0649) (-74.0749, -38.116) (-73.9985, -38.1667) (-73.922, -38.2172) (-73.8455, -38.2674) (-73.7688, -38.3173) (-73.692, -38.3669) (-73.615, -38.4162) (-73.538, -38.4651) (-73.4609, -38.5138) (-73.3836, -38.5622) (-73.3062, -38.6102) (-73.2287, -38.658) (-73.1511, -38.7054) (-73.0734, -38.7525) (-72.9956, -38.7993) (-72.9176, -38.8458) (-72.8396, -38.8919) (-72.7614, -38.9377) (-72.6831, -38.9832) (-72.6047, -39.0284) (-72.5261, -39.0732) (-72.4475, -39.1176) (-72.3687, -39.1617) (-72.2898, -39.2055) (-72.2108, -39.2489) (-72.1317, -39.2919) (-72.0525, -39.3346) (-71.9731, -39.3769) (-71.8936, -39.4188) (-71.814, -39.4603) (-71.7343, -39.5015) (-71.6544, -39.5422) (-71.5745, -39.5826) (-71.5009, -39.6193) (-71.4433, -39.6478) (-71.4017, -39.6682) (-71.3761, -39.6806) (-71.3666, -39.6853) knots -1 -1 -1 -1 -1 -1 -0.985714 -0.971429 -0.957143 -0.942857 -0.928571 -0.914286 -0.9 -0.885714 -0.871429 -0.857143 -0.842857 -0.828571 -0.814286 -0.8 -0.785714 -0.771429 -0.757143 -0.742857 -0.728571 -0.714286 -0.7 -0.685714 -0.671429 -0.657143 -0.642857 -0.628571 -0.614286 -0.6 -0.585714 -0.571429 -0.557143 -0.542857 -0.528571 -0.514286 -0.5 -0.485714 -0.471429 -0.457143 -0.442857 -0.428571 -0.414286 -0.405839 -0.405839 -0.405839 -0.405839 -0.405839 -0.405839
  arc A84 (-71.3666, -39.6853) -> (-71.6006, -40.9824) centre (-2.0032, -52.8695) ccw
  spline S84 degree 5 poles (-71.6006, -40.9824) (-71.6112, -40.9834) (-71.6395, -40.9862) (-71.6856, -40.9907) (-71.7495, -40.9973) (-71.8312, -41.006) (-71.9203, -41.0158) (-72.0094, -41.0261) (-72.0984, -41.0368) (-72.1875, -41.0479) (-72.2767, -41.0594) (-72.3658, -41.0713) (-72.455, -41.0836) (-72.5441, -41.0963) (-72.6333, -41.1093) (-72.7225, -41.1227) (-72.8117, -41.1365) (-72.901, -41.1507) (-72.9902, -41.1652) (-73.0795, -41.1801) (-73.1687, -41.1954) (-73.258, -41.211) (-73.3472, -41.2269) (-73.4365, -41.2432) (-73.5258, -41.2599) (-73.6151, -41.2768) (-73.7044, -41.2942) (-73.7936, -41.3118) (-73.8829, -41.3298) (-73.9722, -41.3481) (-74.0615, -41.3668) (-74.1508, -41.3858) (-74.2401, -41.4051) (-74.3294, -41.4247) (-74.4187, -41.4446) (-74.508, -41.4649) (-74.5973, -41.4854) (-74.6865, -41.5063) (-74.7758, -41.5275) (-74.8651, -41.549) (-74.9543, -41.5708) (-75.0436, -41.5929) (-75.1329, -41.6154) (-75.2042, -41.6335) (-75.2578, -41.6473) (-75.2935, -41.6565) (-75.3113, -41.6612) knots 0.405839 0.405839 0.405839 0.405839 0.405839 0.405839 0.414286 0.428571 0.442857 0.457143 0.471429 0.485714 0.5 0.514286 0.528571 0.542857 0.557143 0.571429 0.585714 0.6 0.614286 0.628571 0.642857 0.657143 0.671429 0.685714 0.7 0.714286 0.728571 0.742857 0.757143 0.771429 0.785714 0.8 0.814286 0.828571 0.842857 0.857143 0.871429 0.885714 0.9 0.914286 0.928571 0.942857 0.957143 0.971429 0.985714 1 1 1 1 1 1
  arc A85 (-75.3113, -41.6612) -> (-75.4996, -42.9705) centre (-2.0032, -52.8695) ccw
  spline S85 degree 5 poles (-75.4996, -42.9705) (-75.4838, -42.98) (-75.4521, -42.9989) (-75.4046, -43.0272) (-75.3412, -43.0647) (-75.2619, -43.1114) (-75.1825, -43.1577) (-75.103, -43.2038) (-75.0234, -43.2496) (-74.9437, -43.2951) (-74.8639, -43.3403) (-74.7841, -43.3852) (-74.7041, -43.4298) (-74.6241, -43.4741) (-74.5439, -43.518) (-74.4637, -43.5617) (-74.3833, -43.6051) (-74.3029, -43.6481) (-74.2224, -43.6909) (-74.1418, -43.7333) (-74.0611, -43.7754) (-73.9803, -43.8172) (-73.8994, -43.8586) (-73.8185, -43.8997) (-73.7374, -43.9405) (-73.6562, -43.981) (-73.575, -44.0211) (-73.4936, -44.0608) (-73.4122, -44.1003) (-73.3307, -44.1394) (-73.2491, -44.1781) (-73.1673, -44.2165) (-73.0855, -44.2545) (-73.0036, -44.2921) (-72.9216, -44.3294) (-72.8396, -44.3663) (-72.7574, -44.4028) (-72.6751, -44.439) (-72.5927, -44.4747) (-72.5103, -44.5101) (-72.4277, -44.5451) (-72.3451, -44.5796) (-72.2691, -44.611) (-72.2096, -44.6353) (-72.1666, -44.6526) (-72.1402, -44.6632) (-72.1304, -44.6672) knots -1 -1 -1 -1 -1 -1 -0.985714 -0.971429 -0.957143 -0.942857 -0.928571 -0.914286 -0.9 -0.885714 -0.871429 -0.857143 -0.842857 -0.828571 -0.814286 -0.8 -0.785714 -0.771429 -0.757143 -0.742857 -0.728571 -0.714286 -0.7 -0.685714 -0.671429 -0.657143 -0.642857 -0.628571 -0.614286 -0.6 -0.585714 -0.571429 -0.557143 -0.542857 -0.528571 -0.514286 -0.5 -0.485714 -0.471429 -0.457143 -0.442857 -0.428571 -0.414286 -0.405839 -0.405839 -0.405839 -0.405839 -0.405839 -0.405839
  arc A86 (-72.1304, -44.6672) -> (-72.2713, -45.9777) centre (-2.0032, -52.8695) ccw
  spline S86 degree 5 poles (-72.2713, -45.9777) (-72.2817, -45.9795) (-72.3098, -45.9843) (-72.3555, -45.9921) (-72.4188, -46.0032) (-72.4997, -46.0177) (-72.5878, -46.0339) (-72.6759, -46.0505) (-72.764, -46.0675) (-72.8521, -46.0849) (-72.9401, -46.1028) (-73.0282, -46.121) (-73.1163, -46.1396) (-73.2043, -46.1586) (-73.2923, -46.178) (-73.3804, -46.1977) (-73.4684, -46.2179) (-73.5563, -46.2384) (-73.6443, -46.2592) (-73.7323, -46.2804) (-73.8202, -46.302) (-73.9081, -46.3239) (-73.996, -46.3462) (-74.0839, -46.3688) (-74.1718, -46.3918) (-74.2596, -46.4151) (-74.3474, -46.4387) (-74.4352, -46.4627) (-74.523, -46.487) (-74.6108, -46.5117) (-74.6985, -46.5367) (-74.7862, -46.562) (-74.8739, -46.5876) (-74.9616, -46.6135) (-75.0492, -46.6398) (-75.1368, -46.6664) (-75.2244, -46.6932) (-75.312, -46.7204) (-75.3995, -46.748) (-75.487, -46.7758) (-75.5745, -46.8039) (-75.662, -46.8323) (-75.7494, -46.861) (-75.8193, -46.8843) (-75.8717, -46.9018) (-75.9067, -46.9136) (-75.9241, -46.9195) knots 0.405839 0.405839 0.405839 0.405839 0.405839 0.405839 0.414286 0.428571 0.442857 0.457143 0.471429 0.485714 0.5 0.514286 0.528571 0.542857 0.557143 0.571429 0.585714 0.6 0.614286 0.628571 0.642857 0.657143 0.671429 0.685714 0.7 0.714286 0.728571 0.742857 0.757143 0.771429 0.785714 0.8 0.814286 0.828571 0.842857 0.857143 0.871429 0.885714 0.9 0.914286 0.928571 0.942857 0.957143 0.971429 0.985714 1 1 1 1 1 1
  arc A87 (-75.9241, -46.9195) -> (-76.0185, -48.2389) centre (-2.0032, -52.8695) ccw
  spline S87 degree 5 poles (-76.0185, -48.2389) (-76.0021, -48.2472) (-75.9691, -48.2638) (-75.9197, -48.2887) (-75.8538, -48.3216) (-75.7714, -48.3625) (-75.6889, -48.403) (-75.6063, -48.4433) (-75.5236, -48.4833) (-75.4409, -48.523) (-75.3581, -48.5624) (-75.2752, -48.6015) (-75.1923, -48.6402) (-75.1093, -48.6787) (-75.0262, -48.7169) (-74.9431, -48.7547) (-74.8598, -48.7922) (-74.7766, -48.8294) (-74.6932, -48.8663) (-74.6098, -48.9029) (-74.5263, -48.9391) (-74.4427, -48.975) (-74.3591, -49.0106) (-74.2754, -49.0458) (-74.1916, -49.0807) (-74.1078, -49.1153) (-74.0239, -49.1495) (-73.9399, -49.1834) (-73.8558, -49.2169) (-73.7717, -49.25) (-73.6876, -49.2828) (-73.6033, -49.3153) (-73.519, -49.3474) (-73.4346, -49.3791) (-73.3502, -49.4104) (-73.2657, -49.4414) (-73.1811, -49.4719) (-73.0965, -49.5021) (-73.0118, -49.5319) (-72.927, -49.5613) (-72.8421, -49.5903) (-72.7572, -49.6189) (-72.6792, -49.6447) (-72.6181, -49.6647) (-72.574, -49.679) (-72.547, -49.6877) (-72.5369, -49.6909) knots -1 -1 -1 -1 -1 -1 -0.985714 -0.971429 -0.957143 -0.942857 -0.928571 -0.914286 -0.9 -0.885714 -0.871429 -0.857143 -0.842857 -0.828571 -0.814286 -0.8 -0.785714 -0.771429 -0.757143 -0.742857 -0.728571 -0.714286 -0.7 -0.685714 -0.671429 -0.657143 -0.642857 -0.628571 -0.614286 -0.6 -0.585714 -0.571429 -0.557143 -0.542857 -0.528571 -0.514286 -0.5 -0.485714 -0.471429 -0.457143 -0.442857 -0.428571 -0.414286 -0.405839 -0.405839 -0.405839 -0.405839 -0.405839 -0.405839
  arc A88 (-72.5369, -49.6909) -> (-72.5839, -51.0082) centre (-2.0032, -52.8695) ccw
  spline S88 degree 5 poles (-72.5839, -51.0082) (-72.5942, -51.0107) (-72.6218, -51.0174) (-72.6668, -51.0285) (-72.7292, -51.044) (-72.8089, -51.0643) (-72.8956, -51.0867) (-72.9823, -51.1096) (-73.0689, -51.1329) (-73.1556, -51.1565) (-73.2421, -51.1806) (-73.3287, -51.2051) (-73.4152, -51.2299) (-73.5016, -51.2551) (-73.5881, -51.2807) (-73.6744, -51.3067) (-73.7608, -51.3331) (-73.8471, -51.3598) (-73.9333, -51.3869) (-74.0196, -51.4143) (-74.1057, -51.4421) (-74.1919, -51.4702) (-74.278, -51.4987) (-74.364, -51.5276) (-74.45, -51.5567) (-74.536, -51.5863) (-74.6219, -51.6161) (-74.7077, -51.6463) (-74.7936, -51.6768) (-74.8793, -51.7077) (-74.9651, -51.7388) (-75.0508, -51.7703) (-75.1364, -51.8021) (-75.222, -51.8343) (-75.3075, -51.8667) (-75.393, -51.8995) (-75.4785, -51.9325) (-75.5639, -51.9659) (-75.6492, -51.9996) (-75.7345, -52.0336) (-75.8198, -52.0679) (-75.905, -52.1025) (-75.9901, -52.1373) (-76.0582, -52.1655) (-76.1092, -52.1867) (-76.1433, -52.201) (-76.1603, -52.2081) knots 0.405839 0.405839 0.405839 0.405839 0.405839 0.405839 0.414286 0.428571 0.442857 0.457143 0.471429 0.485714 0.5 0.514286 0.528571 0.542857 0.557143 0.571429 0.585714 0.6 0.614286 0.628571 0.642857 0.657143 0.671429 0.685714 0.7 0.714286 0.728571 0.742857 0.757143 0.771429 0.785714 0.8 0.814286 0.828571 0.842857 0.857143 0.871429 0.885714 0.9 0.914286 0.928571 0.942857 0.957143 0.971429 0.985714 1 1 1 1 1 1
  arc A89 (-76.1603, -52.2081) -> (-76.1603, -53.5309) centre (-2.0032, -52.8695) ccw
  spline S89 degree 5 poles (-76.1603, -53.5309) (-76.1433, -53.538) (-76.1092, -53.5522) (-76.0582, -53.5735) (-75.9901, -53.6016) (-75.905, -53.6365) (-75.8198, -53.6711) (-75.7345, -53.7054) (-75.6492, -53.7394) (-75.5639, -53.7731) (-75.4785, -53.8064) (-75.393, -53.8395) (-75.3075, -53.8723) (-75.222, -53.9047) (-75.1364, -53.9368) (-75.0508, -53.9686) (-74.9651, -54.0001) (-74.8793, -54.0313) (-74.7936, -54.0621) (-74.7077, -54.0927) (-74.6219, -54.1228) (-74.536, -54.1527) (-74.45, -54.1822) (-74.364, -54.2114) (-74.278, -54.2402) (-74.1919, -54.2687) (-74.1057, -54.2969) (-74.0196, -54.3247) (-73.9333, -54.3521) (-73.8471, -54.3792) (-73.7608, -54.4059) (-73.6744, -54.4322) (-73.5881, -54.4582) (-73.5016, -54.4838) (-73.4152, -54.5091) (-73.3287, -54.5339) (-73.2421, -54.5584) (-73.1556, -54.5824) (-73.0689, -54.6061) (-72.9823, -54.6294) (-72.8956, -54.6522) (-72.8089, -54.6747) (-72.7292, -54.6949) (-72.6668, -54.7105) (-72.6218, -54.7216) (-72.5942, -54.7283) (-72.5839, -54.7308) knots -1 -1 -1 -1 -1 -1 -0.985714 -0.971429 -0.957143 -0.942857 -0.928571 -0.914286 -0.9 -0.885714 -0.871429 -0.857143 -0.842857 -0.828571 -0.814286 -0.8 -0.785714 -0.771429 -0.757143 -0.742857 -0.728571 -0.714286 -0.7 -0.685714 -0.671429 -0.657143 -0.642857 -0.628571 -0.614286 -0.6 -0.585714 -0.571429 -0.557143 -0.542857 -0.528571 -0.514286 -0.5 -0.485714 -0.471429 -0.457143 -0.442857 -0.428571 -0.414286 -0.405839 -0.405839 -0.405839 -0.405839 -0.405839 -0.405839
  arc A90 (-72.5839, -54.7308) -> (-72.5369, -56.0481) centre (-2.0032, -52.8695) ccw
  spline S90 degree 5 poles (-72.5369, -56.0481) (-72.547, -56.0513) (-72.574, -56.06) (-72.6181, -56.0743) (-72.6792, -56.0942) (-72.7572, -56.1201) (-72.8421, -56.1487) (-72.927, -56.1777) (-73.0118, -56.207) (-73.0965, -56.2368) (-73.1811, -56.267) (-73.2657, -56.2976) (-73.3502, -56.3285) (-73.4346, -56.3599) (-73.519, -56.3916) (-73.6033, -56.4237) (-73.6876, -56.4561) (-73.7717, -56.4889) (-73.8558, -56.5221) (-73.9399, -56.5556) (-74.0239, -56.5895) (-74.1078, -56.6237) (-74.1916, -56.6582) (-74.2754, -56.6931) (-74.3591, -56.7284) (-74.4427, -56.764) (-74.5263, -56.7999) (-74.6098, -56.8361) (-74.6932, -56.8727) (-74.7766, -56.9095) (-74.8598, -56.9467) (-74.9431, -56.9843) (-75.0262, -57.0221) (-75.1093, -57.0603) (-75.1923, -57.0987) (-75.2752, -57.1375) (-75.3581, -57.1766) (-75.4409, -57.216) (-75.5236, -57.2556) (-75.6063, -57.2956) (-75.6889, -57.3359) (-75.7714, -57.3765) (-75.8538, -57.4174) (-75.9197, -57.4503) (-75.9691, -57.4751) (-76.0021, -57.4918) (-76.0185, -57.5001) knots 0.405839 0.405839 0.405839 0.405839 0.405839 0.405839 0.414286 0.428571 0.442857 0.457143 0.471429 0.485714 0.5 0.514286 0.528571 0.542857 0.557143 0.571429 0.585714 0.6 0.614286 0.628571 0.642857 0.657143 0.671429 0.685714 0.7 0.714286 0.728571 0.742857 0.757143 0.771429 0.785714 0.8 0.814286 0.828571 0.842857 0.857143 0.871429 0.885714 0.9 0.914286 0.928571 0.942857 0.957143 0.971429 0.985714 1 1 1 1 1 1
  arc A91 (-76.0185, -57.5001) -> (-75.9241, -58.8195) centre (-2.0032, -52.8695) ccw
  spline S91 degree 5 poles (-75.9241, -58.8195) (-75.9067, -58.8254) (-75.8717, -58.8371) (-75.8193, -58.8547) (-75.7494, -58.8779) (-75.662, -58.9066) (-75.5745, -58.9351) (-75.487, -58.9632) (-75.3995, -58.991) (-75.312, -59.0185) (-75.2244, -59.0457) (-75.1368, -59.0726) (-75.0492, -59.0992) (-74.9616, -59.1254) (-74.8739, -59.1514) (-74.7862, -59.177) (-74.6985, -59.2023) (-74.6108, -59.2273) (-74.523, -59.2519) (-74.4352, -59.2762) (-74.3474, -59.3002) (-74.2596, -59.3239) (-74.1718, -59.3472) (-74.0839, -59.3701) (-73.996, -59.3928) (-73.9081, -59.415) (-73.8202, -59.437) (-73.7323, -59.4585) (-73.6443, -59.4798) (-73.5563, -59.5006) (-73.4684, -59.5211) (-73.3804, -59.5412) (-73.2923, -59.561) (-73.2043, -59.5804) (-73.1163, -59.5994) (-73.0282, -59.618) (-72.9401, -59.6362) (-72.8521, -59.654) (-72.764, -59.6715) (-72.6759, -59.6885) (-72.5878, -59.7051) (-72.4997, -59.7213) (-72.4188, -59.7358) (-72.3555, -59.7469) (-72.3098, -59.7547) (-72.2817, -59.7595) (-72.2713, -59.7612) knots -1 -1 -1 -1 -1 -1 -0.985714 -0.971429 -0.957143 -0.942857 -0.928571 -0.914286 -0.9 -0.885714 -0.871429 -0.857143 -0.842857 -0.828571 -0.814286 -0.8 -0.785714 -0.771429 -0.757143 -0.742857 -0.728571 -0.714286 -0.7 -0.685714 -0.671429 -0.657143 -0.642857 -0.628571 -0.614286 -0.6 -0.585714 -0.571429 -0.557143 -0.542857 -0.528571 -0.514286 -0.5 -0.485714 -0.471429 -0.457143 -0.442857 -0.428571 -0.414286 -0.405839 -0.405839 -0.405839 -0.405839 -0.405839 -0.405839
  arc A92 (-72.2713, -59.7612) -> (-72.1304, -61.0718) centre (-2.0032, -52.8695) ccw
  spline S92 degree 5 poles (-72.1304, -61.0718) (-72.1402, -61.0757) (-72.1666, -61.0863) (-72.2096, -61.1037) (-72.2691, -61.128) (-72.3451, -61.1593) (-72.4277, -61.1939) (-72.5103, -61.2289) (-72.5927, -61.2642) (-72.6751, -61.3) (-72.7574, -61.3361) (-72.8396, -61.3727) (-72.9216, -61.4096) (-73.0036, -61.4469) (-73.0855, -61.4845) (-73.1673, -61.5225) (-73.2491, -61.5609) (-73.3307, -61.5996) (-73.4122, -61.6387) (-73.4936, -61.6781) (-73.575, -61.7179) (-73.6562, -61.758) (-73.7374, -61.7985) (-73.8185, -61.8392) (-73.8994, -61.8804) (-73.9803, -61.9218) (-74.0611, -61.9636) (-74.1418, -62.0057) (-74.2224, -62.0481) (-74.3029, -62.0908) (-74.3833, -62.1339) (-74.4637, -62.1773) (-74.5439, -62.2209) (-74.6241, -62.2649) (-74.7041, -62.3092) (-74.7841, -62.3538) (-74.8639, -62.3987) (-74.9437, -62.4439) (-75.0234, -62.4894) (-75.103, -62.5351) (-75.1825, -62.5812) (-75.2619, -62.6276) (-75.3412, -62.6742) (-75.4046, -62.7118) (-75.4521, -62.7401) (-75.4838, -62.759) (-75.4996, -62.7685) knots 0.405839 0.405839 0.405839 0.405839 0.405839 0.405839 0.414286 0.428571 0.442857 0.457143 0.471429 0.485714 0.5 0.514286 0.528571 0.542857 0.557143 0.571429 0.585714 0.6 0.614286 0.628571 0.642857 0.657143 0.671429 0.685714 0.7 0.714286 0.728571 0.742857 0.757143 0.771429 0.785714 0.8 0.814286 0.828571 0.842857 0.857143 0.871429 0.885714 0.9 0.914286 0.928571 0.942857 0.957143 0.971429 0.985714 1 1 1 1 1 1
  arc A93 (-75.4996, -62.7685) -> (-75.3113, -64.0778) centre (-2.0032, -52.8695) ccw
  spline S93 degree 5 poles (-75.3113, -64.0778) (-75.2935, -64.0824) (-75.2578, -64.0917) (-75.2042, -64.1054) (-75.1329, -64.1236) (-75.0436, -64.146) (-74.9543, -64.1681) (-74.8651, -64.1899) (-74.7758, -64.2114) (-74.6865, -64.2326) (-74.5973, -64.2535) (-74.508, -64.2741) (-74.4187, -64.2943) (-74.3294, -64.3143) (-74.2401, -64.3339) (-74.1508, -64.3532) (-74.0615, -64.3722) (-73.9722, -64.3908) (-73.8829, -64.4092) (-73.7936, -64.4271) (-73.7044, -64.4448) (-73.6151, -64.4621) (-73.5258, -64.4791) (-73.4365, -64.4958) (-73.3472, -64.512) (-73.258, -64.528) (-73.1687, -64.5436) (-73.0795, -64.5588) (-72.9902, -64.5737) (-72.901, -64.5883) (-72.8117, -64.6024) (-72.7225, -64.6162) (-72.6333, -64.6296) (-72.5441, -64.6427) (-72.455, -64.6554) (-72.3658, -64.6676) (-72.2767, -64.6795) (-72.1875, -64.691) (-72.0984, -64.7021) (-72.0094, -64.7128) (-71.9203, -64.7231) (-71.8312, -64.733) (-71.7495, -64.7417) (-71.6856, -64.7482) (-71.6395, -64.7528) (-71.6112, -64.7555) (-71.6006, -64.7565) knots -1 -1 -1 -1 -1 -1 -0.985714 -0.971429 -0.957143 -0.942857 -0.928571 -0.914286 -0.9 -0.885714 -0.871429 -0.857143 -0.842857 -0.828571 -0.814286 -0.8 -0.785714 -0.771429 -0.757143 -0.742857 -0.728571 -0.714286 -0.7 -0.685714 -0.671429 -0.657143 -0.642857 -0.628571 -0.614286 -0.6 -0.585714 -0.571429 -0.557143 -0.542857 -0.528571 -0.514286 -0.5 -0.485714 -0.471429 -0.457143 -0.442857 -0.428571 -0.414286 -0.405839 -0.405839 -0.405839 -0.405839 -0.405839 -0.405839
  arc A94 (-71.6006, -64.7565) -> (-71.3666, -66.0537) centre (-2.0032, -52.8695) ccw
  spline S94 degree 5 poles (-71.3666, -66.0537) (-71.3761, -66.0583) (-71.4017, -66.0708) (-71.4433, -66.0912) (-71.5009, -66.1196) (-71.5745, -66.1563) (-71.6544, -66.1967) (-71.7343, -66.2375) (-71.814, -66.2786) (-71.8936, -66.3202) (-71.9731, -66.3621) (-72.0525, -66.4044) (-72.1317, -66.4471) (-72.2108, -66.4901) (-72.2898, -66.5335) (-72.3687, -66.5773) (-72.4475, -66.6214) (-72.5261, -66.6658) (-72.6047, -66.7106) (-72.6831, -66.7557) (-72.7614, -66.8012) (-72.8396, -66.847) (-72.9176, -66.8932) (-72.9956, -66.9396) (-73.0734, -66.9864) (-73.1511, -67.0335) (-73.2287, -67.081) (-73.3062, -67.1287) (-73.3836, -67.1768) (-73.4609, -67.2251) (-73.538, -67.2738) (-73.615, -67.3228) (-73.692, -67.3721) (-73.7688, -67.4217) (-73.8455, -67.4716) (-73.922, -67.5218) (-73.9985, -67.5722) (-74.0749, -67.623) (-74.1511, -67.6741) (-74.2272, -67.7254) (-74.3032, -67.777) (-74.3791, -67.8289) (-74.4549, -67.8811) (-74.5155, -67.9231) (-74.5608, -67.9547) (-74.591, -67.9758) (-74.6061, -67.9864) knots 0.405839 0.405839 0.405839 0.405839 0.405839 0.405839 0.414286 0.428571 0.442857 0.457143 0.471429 0.485714 0.5 0.514286 0.528571 0.542857 0.557143 0.571429 0.585714 0.6 0.614286 0.628571 0.642857 0.657143 0.671429 0.685714 0.7 0.714286 0.728571 0.742857 0.757143 0.771429 0.785714 0.8 0.814286 0.828571 0.842857 0.857143 0.871429 0.885714 0.9 0.914286 0.928571 0.942857 0.957143 0.971429 0.985714 1 1 1 1 1 1